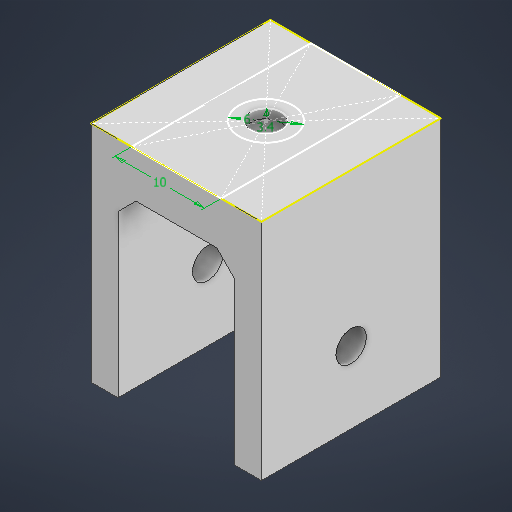
# Autodesk Inventor part: Idlert Tensioner
Saved by Autodesk Inventor 2025.1 (Build 291241000, 241)
## iProperties
Created: 2025-01-23
Part Number: Idlert Tensioner
Material: Generic
Document SubType Name: Modeling
Designer: jerem
Density: 1 g/cm^3
Appearance: Default
Author: jerem
## iProperties of the stored document Idlert Tensioner_3DPrint.ipt
Created: 2025-01-23
Part Number: Idlert Tensioner_3DPrint
Material: Generic
Document SubType Name: Modeling
Designer: jerem
Density: 1 g/cm^3
Appearance: Default
Author: jerem
Autodesk Inventor part; units mm, degrees
ref_plane "YZ Plane" through (0, 0, 0) normal (1, 0, 0) x (0, 1, 0)
ref_plane "XZ Plane" through (0, 0, 0) normal (0, 1, 0) x (-1, 0, 0)
ref_plane "XY Plane" through (0, 0, 0) normal (0, 0, 1) x (1, 0, 0)
sketch "Sketch3" plane through (0, 0, 0) normal (0, 1, 0) x (-1, 0, 0)
  line L0 (-9.5, 10) -> (9.5, 10)
  line L1 (9.5, 10) -> (9.5, -10)
  line L2 (9.5, -10) -> (-9.5, -10)
  line L3 (-9.5, -10) -> (-9.5, 10)
  line L4 (-9.5, 10) -> (9.5, -10) construction
  line L5 (9.5, 10) -> (-9.5, -10) construction
  line L6 (6.5, -10) -> (6.5, 10)
  line L7 (-6.5, 10) -> (-6.5, -10)
  line L8 (-6.5, -6.8421) -> (6.5, -6.8421) construction
  point P0 (0, 0)
  dimension "d12" = 20
  dimension "d17" = 3
  dimension "d36" = 13
  constraints: 18 end point, 8 point on line, 3 perpendicular, 2 horizontal, 2 midpoint, 2 parallel
  measures "d12" distance of L0.end L1.end
  measures "d17" distance between parallel lines of L1 L6
  measures "d36" distance between parallel lines of L7 L6
extrude "Extrusion3" add sketch "Sketch3" along normal blind 25
sketch "Sketch4" plane through (9.5, 0, 10) normal (1, 0, 0) x (0, 0, -1)
  line L0 (10, 0) -> (10, 8) construction
  circle A0 centre (10, 8) radius 1.7
  line L1 (0, 0) -> (20, 0) projected
  dimension "d15" = 3.4
  dimension "d16" = 8
  constraints: 2 end point, 1 centre point, 1 coincident, 1 vertical
  measures "d15" diameter of A0
  measures "d16" distance from line of L1 L0.end
extrude "Extrusion4" cut sketch "Sketch3" along normal blind 20 contours L0 L6 L2 L7
extrude "Extrusion5" cut sketch "Sketch4" against normal through all
sketch "Sketch5" plane through (0, 25, 0) normal (0, 1, 0) x (1, 0, 0)
  line L0 (-6.5, -10) -> (6.5, -10) projected
  line L1 (-5, 10) -> (5, 10)
  line L2 (5, 10) -> (5, -10)
  line L3 (5, -10) -> (-5, -10)
  line L4 (-5, -10) -> (-5, 10)
  line L5 (-5, 10) -> (5, -10) construction
  line L6 (5, 10) -> (-5, -10) construction
  point P0 (0, 0)
  dimension "d22" = 10
  constraints: 12 end point, 2 midpoint, 2 parallel, 1 horizontal, 1 perpendicular, 1 point on line
  measures "d22" distance of L2.end L3.end
sketch "Sketch7" plane through (0, 25, 0) normal (0, 1, 0) x (1, 0, 0)
  circle A0 centre (0, 0) radius 1.7
  circle A1 centre (0, 0) radius 3
  line L0 (-5, 10) -> (5, -10) construction
  line L1 (9.5, 10) -> (-9.5, 10) projected
  line L2 (-9.5, 10) -> (-9.5, -10) projected
  line L3 (-9.5, -10) -> (9.5, -10) projected
  line L4 (9.5, -10) -> (9.5, 10) projected
  line L5 (-9.5, 10) -> (9.5, -10) construction
  line L6 (9.5, 10) -> (-9.5, -10) construction
  dimension "d30" = 3.4
  dimension "d47" = 6
  constraints: 4 end point, 2 centre point, 1 coincident, 1 midpoint
  measures "d30" diameter of A0
  measures "d47" diameter of A1
extrude "Extrusion8" cut sketch "Sketch7" along normal through all both and the other way through all contours A0
chamfer "Chamfer2" distance 2 angle 45 2 edges at (6.5, 20, 0) (-6.5, 20, 0)
extrude "Extrusion9" cut sketch "Sketch7" along normal blind 4 from surface at -5 contours A1
body "Solid2"
